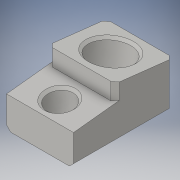
# Autodesk Inventor part: led_holder_v12
Saved by Autodesk Inventor 2016 (Build 200138000, 138)
## iProperties
Created: 2018-09-25
Part Number: led_holder_v12
Material: Generic
Document SubType Name: Modeling
Designer: tar
Density: 1 g/cm^3
Appearance: Default
Author: tar
Autodesk Inventor part; units mm, degrees
ref_plane "YZ Plane" through (0, 0, 0) normal (1, 0, 0) x (0, 1, 0)
ref_plane "XZ Plane" through (0, 0, 0) normal (0, 1, 0) x (-1, 0, 0)
ref_plane "XY Plane" through (0, 0, 0) normal (0, 0, 1) x (1, 0, 0)
sketch "Skizze5" plane through (0, 0, 0) normal (1, 0, 0) x (0, 1, 0)
  line L0 (0, 0) -> (0.5, 0)
  line L1 (0.5, 0) -> (4.9737, 0.486)
  line L2 (4.9737, 0.486) -> (11.4319, -0.2498)
  line L3 (11.4319, -0.2498) -> (11.9319, -0.2498)
  line L4 (11.9319, -0.2498) -> (11.9319, 5.2288)
  line L5 (11.9319, 5.2288) -> (4.9737, 6.0216)
  line L6 (0, 3.4663) -> (0, 0)
  line L7 (0, 3.4663) -> (4.9737, 4.0066)
  line L8 (4.9737, 8.0188) -> (4.9737, 2.9641) construction
  line L9 (4.9737, 6.0216) -> (4.9737, 4.0066)
  point P0 (0, 0)
  dimension "d21" = 0.5
  dimension "d22" = 6.2
  dimension "d23" = 6.5
  dimension "d24" = 4.5
  dimension "d25" = 6.5
  dimension "d26" = 5.5
  dimension "d27" = 3.5
  constraints: 20 end point, 5 point on line, 4 parallel, 2 perpendicular, 1 horizontal, 1 vertical
  measures "d21" distance of L0.start L0.end
  measures "d22" angle of L1 L0
  measures "d23" angle of L2 L3
  measures "d24" distance of L0.end L1.end
  measures "d25" distance of L1.end L2.end
  measures "d26" distance between parallel lines of L5 L2
  measures "d27" distance between parallel lines of L1 L7
extrude "Extrusion3" add sketch "Skizze5" along normal blind 8
sketch "Skizze6" plane through (8, 11.4319, -0.2498) normal (0, -0.1132032, -0.9935719) x (-1, 0, 0)
  circle A0 centre (4, -3.625) radius 2.425
  line L0 (4, 1.7492) -> (4, -8.8787)
  line L1 (-1.2914, -3.625) -> (9.5036, -3.625)
  line L2 (8, -0.1234) -> (8, -7.1266) projected
  line L3 (8, 0.4968) -> (0, 0.4968) projected
  point P0 (8, -11.3867)
  point P1 (8, -3.625)
  point P2 (4, 0.4968)
  dimension "d30" = 4.85
  constraints: 4 end point, 4 point on line, 2 midpoint, 1 centre point, 1 horizontal, 1 vertical
  measures "d30" diameter of A0
extrude "Extrusion4" cut sketch "Skizze6" against normal through all
sketch "Skizze7" plane through (8, 4.9737, 0.486) normal (0, 0.1079994, -0.994151) x (-1, 0, 0)
  line L0 (-0.408, -2.25) -> (9.5226, -2.25)
  line L1 (4, -0.248) -> (4, -7.2475)
  line L2 (8, -4.9971) -> (0, -4.9971) projected
  line L3 (8, -4.5) -> (8, 0) projected
  circle A0 centre (4, -2.25) radius 1.575
  point P0 (4, -4.9971)
  point P1 (8, -2.25)
  dimension "d33" = 3.15
  constraints: 4 end point, 4 point on line, 2 midpoint, 1 centre point, 1 horizontal, 1 vertical
  measures "d33" diameter of A0
extrude "Extrusion5" cut sketch "Skizze7" against normal through all
sketch "Skizze8" plane through (0, 11.4319, -0.2498) normal (0, 0, -1) x (-1, 0, 0)
  line L0 (-8, -6.4582) -> (-8, 0) projected
  line L1 (-8, -10.9319) -> (-8, -6.4582) projected
  line L2 (-8, -11.4319) -> (-8, -10.9319) projected
  line L3 (0, -11.4319) -> (-8, -11.4319) projected
  line L4 (0, -11.4319) -> (0, -10.9319) projected
  line L5 (0, -10.9319) -> (0, -6.4582) projected
  line L6 (0, -6.4582) -> (0, 0) projected
  line L7 (0, 0) -> (0, 0.5) projected
  line L8 (0, 0.5) -> (-8, 0.5) projected
  line L9 (-8, 0) -> (-8, 0.5) projected
extrude "Extrusion6" add sketch "Skizze8" against normal blind 0.75
sketch "Skizze9" plane through (0, 4.9737, 6.0216) normal (0, 0.1132032, 0.9935719) x (1, 0, 0)
  circle A0 centre (4, 3.5016) radius 2.425 projected
  point P0 (0, -4.26)
extrude "Extrusion7" cut sketch "Skizze9" against normal through all
sketch "Skizze10" plane through (0, 0, 3.4663) normal (0, -0.1079994, 0.994151) x (1, 0, 0)
  circle A0 centre (4, 2.3727) radius 1.575 projected
  point P0 (0, -0.3744)
extrude "Extrusion8" cut sketch "Skizze10" against normal through all
chamfer "Fase2" distance 0.5 angle 45 7 edges at (8, 5.9659, -0.2498) (4, 11.9319, -0.2498) (8, 11.9319, 2.4895) (0, 5.9659, -0.2498) (0, 11.9319, 2.4895) (8, 4.9737, 5.0141) (0, 4.9737, 5.0141)
chamfer "Fase3" distance 0.3 angle 45 2 edges at (6.425, 8.4528, 5.6252) (5.575, 2.3588, 3.7225)
